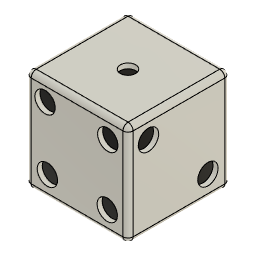
Exercice Formation (Dé 3D) v1 (Autodesk Fusion 360 design; units mm, degrees)
Autodesk Fusion 360 part; units mm, degrees
sketch "Esquisse2" plane through (0, 0, 0) normal (0, 1, 0) x (1, 0, 0)
sketch "Esquisse4" plane through (0, 0, 0) normal (0, 0, 1) x (1, 0, 0)
  line L0 (-4.9636, 6.991) -> (15.0364, 6.991)
  line L1 (15.0364, 6.991) -> (15.0364, -13.009)
  line L2 (15.0364, -13.009) -> (-4.9636, -13.009)
  line L3 (-4.9636, -13.009) -> (-4.9636, 6.991)
  dimension "d9" = 20
  dimension "d10" = 20
  constraint horizontal L0
  constraint vertical L1
  constraint horizontal L2
  constraint vertical L3
  measures "d9" distance of L1 L3
  measures "d10" distance of L0.end L1.end
extrude "Extrusion1" add sketch "Esquisse4" along normal blind 20
sketch "Esquisse5" plane through (0, 0, 20) normal (0, 0, 1) x (-1, 0, 0)
  line L0 (4.9636, 13.009) -> (-15.0364, 13.009)
  line L1 (-15.0364, 13.009) -> (-15.0364, -6.991)
  line L2 (-15.0364, -6.991) -> (4.9636, -6.991)
  line L3 (4.9636, -6.991) -> (4.9636, 13.009)
  circle A0 centre (-5.0364, 3.009) radius 1.5
  line L4 (-15.0364, 13.009) -> (4.9636, -6.991) construction
  dimension "d15" = 3
  constraint coincident L0.end L1.start
  constraint coincident L2.end L3.start
  constraint midpoint A0.centre L4
  measures "d15" diameter of A0
extrude "Extrusion2" cut sketch "Esquisse5" against normal blind 1 contours A0
sketch "Esquisse6" plane through (0, 6.991, 0) normal (0, 1, 0) x (-1, 0, 0)
  line L0 (-15.0364, 0) -> (4.9636, 0)
  line L1 (4.9636, 0) -> (4.9636, 20)
  line L2 (4.9636, 20) -> (-15.0364, 20)
  line L3 (-15.0364, 20) -> (-15.0364, 0)
  line L4 (-15.0364, 20) -> (4.9636, 0) construction
  line L5 (4.9636, 20) -> (-15.0364, 0) construction
  circle A0 centre (-5.1366, 10.1002) radius 1.877
  circle A1 centre (0.9787, 3.9849) radius 2
  circle A2 centre (-11.2908, 16.2544) radius 2
  line L6 (-11.2908, 16.2544) -> (-5.1366, 10.1002) construction
  line L7 (-5.1366, 10.1002) -> (0.9787, 3.9849) construction
  dimension "d16" = 4
  dimension "d17" = 4
  constraint coincident L2.end L3.start
  constraint coincident L0.end L1.start
  constraint coincident L1.end L2.start
  constraint coincident L0.start L3.end
  constraint coincident L4 A0.centre
  constraint coincident L4 A1.centre
  constraint coincident L4 A2.centre
  constraint coincident A2.centre L6.start
  constraint coincident A0.centre L6.end
  constraint coincident A1.centre L7.end
  measures "d16" diameter of A1
  measures "d17" diameter of A2
extrude "Extrusion3" cut sketch "Esquisse6" against normal blind 1 contours A0 | A1 | A2
sketch "Esquisse7" plane through (-4.9636, 0, 0) normal (-1, 0, 0) x (0, -1, 0)
  line L0 (-6.991, 0) -> (13.009, 0)
  line L1 (13.009, 0) -> (13.009, 20)
  line L2 (13.009, 20) -> (-6.991, 20)
  line L3 (-6.991, 20) -> (-6.991, 0)
  line L4 (-6.991, 20) -> (13.009, 0) construction
  line L5 (13.009, 20) -> (-6.991, 0) construction
  circle A0 centre (3.009, 10) radius 2
  circle A1 centre (-3.4749, 16.4839) radius 2
  circle A2 centre (9.2603, 3.7487) radius 2
  circle A3 centre (9.4496, 16.4405) radius 2
  circle A4 centre (-3.4075, 3.5835) radius 2
  dimension "d20" = 4
  dimension "d21" = 4
  dimension "d22" = 4
  dimension "d23" = 4
  dimension "d24" = 4
  constraint coincident L2.end L3.start
  constraint coincident L0.end L1.start
  constraint coincident L1.end L2.start
  constraint coincident L0.start L3.end
  constraint coincident L4 A0.centre
  constraint midpoint L4 A0.centre
  constraint coincident L4 A1.centre
  constraint coincident L4 A2.centre
  constraint coincident L5 A3.centre
  constraint coincident L5 A4.centre
  measures "d20" diameter of A0
  measures "d21" diameter of A1
  measures "d22" diameter of A2
  measures "d23" diameter of A3
  measures "d24" diameter of A4
extrude "Extrusion4" cut sketch "Esquisse7" against normal blind 1 contours A0 | A1 | A2 | A3 | A4
sketch "Esquisse8" plane through (0, 0, 0) normal (0, 0, -1) x (1, 0, 0)
  line L0 (15.0364, 13.009) -> (-4.9636, 13.009)
  line L1 (-4.9636, 13.009) -> (-4.9636, -6.991)
  line L2 (-4.9636, -6.991) -> (15.0364, -6.991)
  line L3 (15.0364, -6.991) -> (15.0364, 13.009)
  line L4 (-4.9636, 13.009) -> (15.0364, -6.991) construction
  line L5 (15.0364, 13.009) -> (-4.9636, -6.991) construction
  circle A0 centre (10.95, -2.9046) radius 2
  circle A1 centre (11.0493, 9.022) radius 2
  circle A2 centre (10.9398, 3.0285) radius 2
  circle A3 centre (-0.8642, 8.9096) radius 2
  circle A4 centre (-1.2323, -3.2596) radius 2
  circle A5 centre (-0.9381, 3.037) radius 2
  dimension "d27" = 4
  dimension "d28" = 4
  dimension "d29" = 4
  dimension "d30" = 4
  dimension "d31" = 4
  dimension "d32" = 4
  constraint coincident L0.end L1.start
  constraint coincident L2.end L3.start
  constraint coincident L0.start L3.end
  constraint coincident L1.end L2.start
  constraint coincident L4 A0.centre
  constraint coincident L5 A1.centre
  constraint coincident L4 A3.centre
  constraint coincident L5 A4.centre
  measures "d27" diameter of A0
  measures "d28" diameter of A1
  measures "d29" diameter of A2
  measures "d30" diameter of A3
  measures "d31" diameter of A4
  measures "d32" diameter of A5
extrude "Extrusion5" cut sketch "Esquisse8" against normal blind 1 contours A0 | A1 | A2 | A3 | A4 | A5
sketch "Esquisse9" plane through (0, -13.009, 0) normal (0, -1, 0) x (1, 0, 0)
  line L0 (-4.9636, 0) -> (15.0364, 0)
  line L1 (15.0364, 0) -> (15.0364, 20)
  line L2 (15.0364, 20) -> (-4.9636, 20)
  line L3 (-4.9636, 20) -> (-4.9636, 0)
  line L4 (-4.9636, 20) -> (15.0364, 0) construction
  line L5 (15.0364, 20) -> (-4.9636, 0) construction
  circle A0 centre (11.0636, 16.0272) radius 2
  circle A1 centre (10.9669, 4.0694) radius 2
  circle A2 centre (-1.2383, 16.2746) radius 2
  circle A3 centre (-0.7874, 4.1763) radius 2
  dimension "d35" = 4
  dimension "d36" = 4
  dimension "d37" = 4
  dimension "d38" = 4
  constraint coincident L2.end L3.start
  constraint coincident L0.end L1.start
  constraint coincident L1.end L2.start
  constraint coincident L0.start L3.end
  constraint coincident L5 A0.centre
  constraint coincident L4 A1.centre
  constraint coincident L4 A2.centre
  constraint coincident L5 A3.centre
  measures "d35" diameter of A0
  measures "d36" diameter of A1
  measures "d37" diameter of A2
  measures "d38" diameter of A3
extrude "Extrusion6" cut sketch "Esquisse9" against normal blind 1 contours A0 | A1 | A2 | A3
sketch "Esquisse10" plane through (15.0364, 0, 0) normal (1, 0, 0) x (0, 1, 0)
  line L0 (-13.009, 0) -> (6.991, 0)
  line L1 (6.991, 0) -> (6.991, 20)
  line L2 (6.991, 20) -> (-13.009, 20)
  line L3 (-13.009, 20) -> (-13.009, 0)
  line L4 (-13.009, 20) -> (6.991, 0) construction
  line L5 (6.991, 20) -> (-13.009, 0) construction
  circle A0 centre (-8.9924, 15.9834) radius 2
  circle A1 centre (2.6774, 4.3136) radius 2
  dimension "d41" = 4
  dimension "d42" = 4
  constraint coincident L2.end L3.start
  constraint coincident L0.end L1.start
  constraint coincident L1.end L2.start
  constraint coincident L0.start L3.end
  constraint coincident L4 A0.centre
  constraint coincident L4 A1.centre
  measures "d41" diameter of A0
  measures "d42" diameter of A1
extrude "Extrusion7" cut sketch "Esquisse10" against normal blind 1 contours A0 | A1
fillet "Congé2" radius 1 12 edges at (15.0364, -3.009, 0) (5.0364, -13.009, 0) (-4.9636, -3.009, 0) (5.0364, 6.991, 0) (15.0364, -13.009, 10) (-4.9636, -13.009, 10) (5.0364, -13.009, 20) (15.0364, -3.009, 20) (15.0364, 6.991, 10) (5.0364, 6.991, 20) (-4.9636, 6.991, 10) (-4.9636, -3.009, 20)
fillet "Congé1" [suppressed]
named bodies: "Corps"
